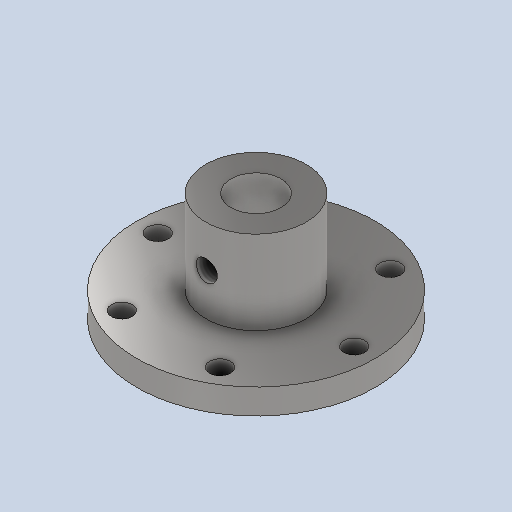
# Autodesk Inventor part: frange
Saved by Autodesk Inventor 2025.1 (Build 291241000, 241)
## iProperties
Created: 2023-11-21
Part Number: frange
Material: ステンレス鋼
Document SubType Name: Modeling
Designer: fhbdh
Density: 8 g/cm^3
Appearance: 半つや出し
Author: fhbdh
Autodesk Inventor part; units mm, degrees
ref_plane "YZ Plane" through (0, 0, 0) normal (1, 0, 0) x (0, 1, 0)
ref_plane "XZ Plane" through (0, 0, 0) normal (0, 1, 0) x (-1, 0, 0)
sketch "スケッチ1" plane through (0, 0, 0) normal (0, 1, 0) x (-1, 0, 0)
  circle A0 centre (0, 0) radius 28.5
  line L0 (-28.5, 0) -> (28.5, 0) construction
  circle A1 centre (23.5, 0) radius 2.5
  circle A2 centre (11.75, 20.3516) radius 2.5
  circle A3 centre (-11.75, 20.3516) radius 2.5
  circle A4 centre (-23.5, 0) radius 2.5
  circle A5 centre (-11.75, -20.3516) radius 2.5
  circle A6 centre (11.75, -20.3516) radius 2.5
  circle A7 centre (0, 0) radius 6
  dimension "d0" = 57
  dimension "d1" = 5
  dimension "d2" = 23.5
  dimension "d6" = 360
  dimension "d10" = 12
  constraints: 8 centre point, 2 coincident, 2 end point, 2 midpoint, 2 point on circle, 1 horizontal, 1 point on line, 13 other
  measures "d0" diameter of A0
  measures "d1" diameter of A1
  measures "d2" distance of point (0, 0) A1.centre
  measures "d10" diameter of A7
extrude "押し出し1" add sketch "スケッチ1" along normal blind 6
sketch "スケッチ2" plane through (0, 6, 0) normal (0, 1, 0) x (1, 0, 0)
  circle A0 centre (0, 0) radius 12
  circle A1 centre (0, 0) radius 6 projected
  dimension "d11" = 24
  constraints: 1 centre point, 1 coincident
  measures "d11" diameter of A0
extrude "押し出し2" add sketch "スケッチ2" along normal blind 20
ref_plane "作業平面1" through (0, 6, 12) normal (0, 0, 1) x (1, 0, 0)
sketch "スケッチ3" plane through (0, 6, 12) normal (0, 0, 1) x (1, 0, 0)
  line L0 (12, 20) -> (-12, 20) projected
  line L1 (12, 20) -> (-12, 20) projected
  line L2 (-12, 0) -> (12, 0) projected
  circle A0 centre (0, 10) radius 2.5
  line L3 (0, 0) -> (0, 20) construction
  point P0 (0, -6)
  dimension "d14" = 20
  dimension "d15" = 5
  dimension "d16" = 10
  constraints: 3 midpoint, 2 end point, 1 centre point
  measures "d14" distance between parallel lines of L2 L0
  measures "d15" diameter of A0
  measures "d16" distance from line of L0 A0.centre
extrude "押し出し3" cut sketch "スケッチ3" against normal up to surface
thread "ねじ1" size "M5x0.8" class "6H" standard "ANSI Metric M Profile" length 55
equation "\"d16\" = 0.5 * d14"
